Autodesk Fusion 360 part; units mm, degrees
note: some values were not read from the file. Set by a fixed rule: which sketch regions a step uses.
(part 15 of 20)
  spline S84 degree 5 poles (-28.7753, 3.9508) (-28.7754, 3.9508) (-28.7756, 3.9508) (-28.7759, 3.9509) (-28.7764, 3.9509) (-28.7772, 3.951) (-28.778, 3.9511) (-28.779, 3.9512) (-28.7801, 3.9514) (-28.7813, 3.9515) (-28.7826, 3.9517) (-28.784, 3.9518) (-28.7855, 3.952) (-28.7871, 3.9522) (-28.7889, 3.9523) (-28.7907, 3.9525) (-28.7926, 3.9527) (-28.7946, 3.9529) (-28.7968, 3.9531) (-28.799, 3.9534) (-28.8013, 3.9536) (-28.8037, 3.9538) (-28.8063, 3.954) (-28.8089, 3.9543) (-28.8116, 3.9545) (-28.8144, 3.9547) (-28.8172, 3.955) (-28.8202, 3.9552) (-28.8233, 3.9555) (-28.8264, 3.9557) (-28.8297, 3.9559) (-28.833, 3.9562) (-28.8364, 3.9564) (-28.8399, 3.9567) (-28.8435, 3.9569) (-28.8472, 3.9572) (-28.8509, 3.9574) (-28.8547, 3.9577) (-28.8586, 3.9579) (-28.8626, 3.9581) (-28.8667, 3.9584) (-28.8709, 3.9586) (-28.8751, 3.9588) (-28.8794, 3.959) (-28.8838, 3.9593) (-28.8882, 3.9595) (-28.8928, 3.9597) (-28.8974, 3.9599) (-28.9021, 3.9601) (-28.9068, 3.9603) (-28.9117, 3.9605) (-28.9166, 3.9607) (-28.9215, 3.9609) (-28.9266, 3.961) (-28.9317, 3.9612) (-28.9369, 3.9614) (-28.9422, 3.9615) (-28.9475, 3.9617) (-28.9529, 3.9618) (-28.9584, 3.962) (-28.9639, 3.9621) (-28.9695, 3.9622) (-28.9752, 3.9623) (-28.9809, 3.9624) (-28.9867, 3.9625) (-28.9926, 3.9626) (-28.9985, 3.9627) (-29.0045, 3.9627) (-29.0106, 3.9628) (-29.0167, 3.9629) (-29.0229, 3.9629) (-29.0291, 3.9629) (-29.0355, 3.9629) (-29.0418, 3.963) (-29.0483, 3.963) (-29.0548, 3.9629) (-29.0613, 3.9629) (-29.068, 3.9629) (-29.0746, 3.9628) (-29.0814, 3.9628) (-29.0882, 3.9627) (-29.095, 3.9626) (-29.1019, 3.9626) (-29.1089, 3.9625) (-29.1159, 3.9623) (-29.123, 3.9622) (-29.1302, 3.9621) (-29.1374, 3.9619) (-29.1446, 3.9618) (-29.1519, 3.9616) (-29.1593, 3.9614) (-29.1667, 3.9612) (-29.1742, 3.961) (-29.1817, 3.9607) (-29.1893, 3.9605) (-29.197, 3.9603) (-29.2047, 3.96) (-29.2124, 3.9597) (-29.2202, 3.9594) (-29.2281, 3.9591) (-29.236, 3.9588) (-29.2439, 3.9584) (-29.2519, 3.9581) (-29.26, 3.9577) (-29.2681, 3.9573) (-29.2763, 3.9569) (-29.2845, 3.9565) (-29.2927, 3.9561) (-29.301, 3.9556) (-29.3094, 3.9552) (-29.3178, 3.9547) (-29.3263, 3.9542) (-29.3348, 3.9537) (-29.3433, 3.9532) (-29.3519, 3.9526) (-29.3606, 3.9521) (-29.3693, 3.9515) (-29.378, 3.9509) (-29.3868, 3.9503) (-29.3957, 3.9497) (-29.4045, 3.9491) (-29.4135, 3.9484) (-29.4225, 3.9478) (-29.4315, 3.9471) (-29.4406, 3.9464) (-29.4497, 3.9457) (-29.4588, 3.9449) (-29.468, 3.9442) (-29.4773, 3.9434) (-29.4866, 3.9426) (-29.4959, 3.9418) (-29.5053, 3.941) (-29.5147, 3.9402) (-29.5242, 3.9393) (-29.5337, 3.9384) (-29.5433, 3.9375) (-29.5529, 3.9366) (-29.5625, 3.9357) (-29.5722, 3.9348) (-29.5819, 3.9338) (-29.5917, 3.9328) (-29.6015, 3.9318) (-29.6113, 3.9308) (-29.6212, 3.9297) (-29.6312, 3.9287) (-29.6411, 3.9276) (-29.6512, 3.9265) (-29.6612, 3.9254) (-29.6713, 3.9243) (-29.6814, 3.9231) (-29.6916, 3.922) (-29.7018, 3.9208) (-29.7121, 3.9196) (-29.7224, 3.9183) (-29.7327, 3.9171) (-29.7431, 3.9158) (-29.7535, 3.9145) (-29.764, 3.9132) (-29.7744, 3.9119) (-29.785, 3.9106) (-29.7955, 3.9092) (-29.8061, 3.9078) (-29.8168, 3.9064) (-29.8274, 3.905) (-29.8382, 3.9035) (-29.8489, 3.9021) (-29.8597, 3.9006) (-29.8705, 3.8991) (-29.8814, 3.8976) (-29.8923, 3.896) (-29.9032, 3.8945) (-29.9142, 3.8929) (-29.9252, 3.8913) (-29.9362, 3.8896) (-29.9473, 3.888) (-29.9584, 3.8863) (-29.9696, 3.8846) (-29.9807, 3.8829) (-29.992, 3.8812) (-30.0032, 3.8795) (-30.0145, 3.8777) (-30.0258, 3.8759) (-30.0372, 3.8741) (-30.0486, 3.8722) (-30.06, 3.8704) (-30.0714, 3.8685) (-30.0829, 3.8666) (-30.0944, 3.8647) (-30.106, 3.8628) (-30.1176, 3.8608) (-30.1292, 3.8588) (-30.1409, 3.8568) (-30.1525, 3.8548) (-30.1643, 3.8527) (-30.176, 3.8507) (-30.1878, 3.8486) (-30.1996, 3.8464) (-30.2115, 3.8443) (-30.2233, 3.8422) (-30.2353, 3.84) (-30.2472, 3.8378) (-30.2592, 3.8356) (-30.2712, 3.8333) (-30.2832, 3.831) (-30.2953, 3.8288) (-30.3074, 3.8264) (-30.3195, 3.8241) (-30.3317, 3.8217) (-30.3439, 3.8194) (-30.3561, 3.817) (-30.3683, 3.8145) (-30.3806, 3.8121) (-30.3929, 3.8096) (-30.4053, 3.8071) (-30.4176, 3.8046) (-30.43, 3.8021) (-30.4424, 3.7995) (-30.4549, 3.797) (-30.4674, 3.7943) (-30.4799, 3.7917) (-30.4924, 3.7891) (-30.505, 3.7864) (-30.5176, 3.7837) (-30.5302, 3.781) (-30.5429, 3.7782) (-30.5556, 3.7755) (-30.5683, 3.7727) (-30.581, 3.7699) (-30.5938, 3.767) (-30.6066, 3.7642) (-30.6194, 3.7613) (-30.6323, 3.7584) (-30.6451, 3.7555) (-30.658, 3.7525) (-30.671, 3.7496) (-30.6839, 3.7466) (-30.6969, 3.7435) (-30.7099, 3.7405) (-30.723, 3.7374) (-30.736, 3.7343) (-30.7491, 3.7312) (-30.7596, 3.7287) (-30.7675, 3.7268) (-30.7728, 3.7256) (-30.7754, 3.7249) knots 0 0 0 0 0 0 0.00416667 0.00833333 0.0125 0.01666667 0.02083333 0.025 0.02916667 0.03333333 0.0375 0.04166667 0.04583333 0.05 0.05416667 0.05833333 0.0625 0.06666667 0.07083333 0.075 0.07916667 0.08333333 0.0875 0.09166667 0.09583333 0.1 0.10416667 0.10833333 0.1125 0.11666667 0.12083333 0.125 0.12916667 0.13333333 0.1375 0.14166667 0.14583333 0.15 0.15416667 0.15833333 0.1625 0.16666667 0.17083333 0.175 0.17916667 0.18333333 0.1875 0.19166667 0.19583333 0.2 0.20416667 0.20833333 0.2125 0.21666667 0.22083333 0.225 0.22916667 0.23333333 0.2375 0.24166667 0.24583333 0.25 0.25416667 0.25833333 0.2625 0.26666667 0.27083333 0.275 0.27916667 0.28333333 0.2875 0.29166667 0.29583333 0.3 0.30416667 0.30833333 0.3125 0.31666667 0.32083333 0.325 0.32916667 0.33333333 0.3375 0.34166667 0.34583333 0.35 0.35416667 0.35833333 0.3625 0.36666667 0.37083333 0.375 0.37916667 0.38333333 0.3875 0.39166667 0.39583333 0.4 0.40416667 0.40833333 0.4125 0.41666667 0.42083333 0.425 0.42916667 0.43333333 0.4375 0.44166667 0.44583333 0.45 0.45416667 0.45833333 0.4625 0.46666667 0.47083333 0.475 0.47916667 0.48333333 0.4875 0.49166667 0.49583333 0.5 0.50416667 0.50833333 0.5125 0.51666667 0.52083333 0.525 0.52916667 0.53333333 0.5375 0.54166667 0.54583333 0.55 0.55416667 0.55833333 0.5625 0.56666667 0.57083333 0.575 0.57916667 0.58333333 0.5875 0.59166667 0.59583333 0.6 0.60416667 0.60833333 0.6125 0.61666667 0.62083333 0.625 0.62916667 0.63333333 0.6375 0.64166667 0.64583333 0.65 0.65416667 0.65833333 0.6625 0.66666667 0.67083333 0.675 0.67916667 0.68333333 0.6875 0.69166667 0.69583333 0.7 0.70416667 0.70833333 0.7125 0.71666667 0.72083333 0.725 0.72916667 0.73333333 0.7375 0.74166667 0.74583333 0.75 0.75416667 0.75833333 0.7625 0.76666667 0.77083333 0.775 0.77916667 0.78333333 0.7875 0.79166667 0.79583333 0.8 0.80416667 0.80833333 0.8125 0.81666667 0.82083333 0.825 0.82916667 0.83333333 0.8375 0.84166667 0.84583333 0.85 0.85416667 0.85833333 0.8625 0.86666667 0.87083333 0.875 0.87916667 0.88333333 0.8875 0.89166667 0.89583333 0.9 0.90416667 0.90833333 0.9125 0.91666667 0.92083333 0.925 0.92916667 0.93333333 0.9375 0.94166667 0.94583333 0.95 0.95416667 0.95833333 0.9625 0.96666667 0.97083333 0.975 0.97916667 0.98333333 0.9875 0.99166667 0.99583333 1 1 1 1 1 1
  arc A83 (-30.9962, 0.4876) -> (-30.9962, -0.4876) centre (0, 0) ccw
  line L180 (-27.8945, 8.0948) -> (-27.8937, 8.0945)
  spline S85 degree 5 poles (12.1618, 28.5147) (12.16, 28.5128) (12.1562, 28.5089) (12.1506, 28.503) (12.1432, 28.4951) (12.134, 28.4854) (12.1248, 28.4756) (12.1156, 28.4658) (12.1065, 28.4561) (12.0973, 28.4464) (12.0883, 28.4366) (12.0792, 28.4269) (12.0702, 28.4172) (12.0613, 28.4075) (12.0523, 28.3978) (12.0434, 28.3882) (12.0345, 28.3785) (12.0257, 28.3689) (12.0169, 28.3593) (12.0081, 28.3496) (11.9994, 28.34) (11.9907, 28.3305) (11.982, 28.3209) (11.9734, 28.3113) (11.9648, 28.3018) (11.9562, 28.2922) (11.9477, 28.2827) (11.9392, 28.2732) (11.9307, 28.2637) (11.9223, 28.2542) (11.9139, 28.2447) (11.9055, 28.2353) (11.8972, 28.2259) (11.8889, 28.2164) (11.8807, 28.207) (11.8724, 28.1976) (11.8643, 28.1882) (11.8561, 28.1789) (11.848, 28.1695) (11.8399, 28.1602) (11.8318, 28.1509) (11.8238, 28.1416) (11.8158, 28.1323) (11.8079, 28.123) (11.8, 28.1137) (11.7921, 28.1045) (11.7843, 28.0953) (11.7765, 28.0861) (11.7687, 28.0769) (11.7609, 28.0677) (11.7532, 28.0585) (11.7456, 28.0494) (11.7379, 28.0403) (11.7303, 28.0312) (11.7228, 28.0221) (11.7153, 28.013) (11.7078, 28.0039) (11.7003, 27.9949) (11.6929, 27.9859) (11.6855, 27.9769) (11.6781, 27.9679) (11.6708, 27.9589) (11.6635, 27.95) (11.6563, 27.9411) (11.6491, 27.9322) (11.6419, 27.9233) (11.6348, 27.9144) (11.6276, 27.9055) (11.6206, 27.8967) (11.6135, 27.8879) (11.6065, 27.8791) (11.5996, 27.8704) (11.5927, 27.8616) (11.5858, 27.8529) (11.5789, 27.8442) (11.5721, 27.8355) (11.5653, 27.8268) (11.5585, 27.8182) (11.5518, 27.8096) (11.5452, 27.801) (11.5385, 27.7924) (11.5319, 27.7838) (11.5253, 27.7753) (11.5188, 27.7668) (11.5123, 27.7583) (11.5058, 27.7498) (11.4994, 27.7414) (11.493, 27.733) (11.4867, 27.7246) (11.4803, 27.7162) (11.4741, 27.7078) (11.4678, 27.6995) (11.4616, 27.6912) (11.4554, 27.6829) (11.4493, 27.6747) (11.4432, 27.6665) (11.4371, 27.6582) (11.4311, 27.6501) (11.4251, 27.6419) (11.4192, 27.6338) (11.4132, 27.6257) (11.4074, 27.6176) (11.4015, 27.6096) (11.3957, 27.6015) (11.3899, 27.5936) (11.3842, 27.5856) (11.3785, 27.5776) (11.3728, 27.5697) (11.3672, 27.5618) (11.3616, 27.554) (11.3561, 27.5462) (11.3506, 27.5384) (11.3451, 27.5306) (11.3396, 27.5228) (11.3342, 27.5151) (11.3289, 27.5074) (11.3235, 27.4998) (11.3183, 27.4922) (11.313, 27.4846) (11.3078, 27.477) (11.3026, 27.4695) (11.2975, 27.462) (11.2924, 27.4545) (11.2873, 27.447) (11.2823, 27.4396) (11.2773, 27.4323) (11.2723, 27.4249) (11.2674, 27.4176) (11.2625, 27.4103) (11.2577, 27.4031) (11.2529, 27.3958) (11.2481, 27.3887) (11.2434, 27.3815) (11.2387, 27.3744) (11.234, 27.3673) (11.2294, 27.3603) (11.2248, 27.3533) (11.2203, 27.3463) (11.2158, 27.3393) (11.2113, 27.3324) (11.2069, 27.3256) (11.2025, 27.3187) (11.1982, 27.3119) (11.1939, 27.3052) (11.1896, 27.2985) (11.1854, 27.2918) (11.1812, 27.2851) (11.177, 27.2785) (11.1729, 27.272) (11.1688, 27.2654) (11.1648, 27.259) (11.1608, 27.2525) (11.1568, 27.2461) (11.1529, 27.2397) (11.149, 27.2334) (11.1451, 27.2271) (11.1413, 27.2209) (11.1376, 27.2147) (11.1338, 27.2085) (11.1301, 27.2024) (11.1265, 27.1963) (11.1229, 27.1903) (11.1193, 27.1843) (11.1158, 27.1784) (11.1123, 27.1725) (11.1088, 27.1666) (11.1054, 27.1608) (11.102, 27.155) (11.0987, 27.1493) (11.0954, 27.1436) (11.0921, 27.138) (11.0889, 27.1324) (11.0857, 27.1269) (11.0826, 27.1214) (11.0795, 27.116) (11.0764, 27.1106) (11.0734, 27.1053) (11.0704, 27.1) (11.0675, 27.0948) (11.0646, 27.0896) (11.0617, 27.0845) (11.0589, 27.0794) (11.0561, 27.0744) (11.0534, 27.0694) (11.0507, 27.0645) (11.048, 27.0597) (11.0454, 27.0549) (11.0428, 27.0501) (11.0403, 27.0454) (11.0378, 27.0408) (11.0353, 27.0362) (11.0329, 27.0317) (11.0306, 27.0272) (11.0282, 27.0228) (11.0259, 27.0185) (11.0237, 27.0142) (11.0215, 27.01) (11.0193, 27.0058) (11.0172, 27.0017) (11.0151, 26.9977) (11.0131, 26.9937) (11.0111, 26.9898) (11.0091, 26.986) (11.0072, 26.9822) (11.0053, 26.9785) (11.0035, 26.9748) (11.0017, 26.9713) (10.9999, 26.9678) (10.9982, 26.9643) (10.9966, 26.961) (10.9949, 26.9577) (10.9934, 26.9544) (10.9918, 26.9513) (10.9903, 26.9482) (10.9889, 26.9452) (10.9875, 26.9423) (10.9861, 26.9394) (10.9848, 26.9366) (10.9835, 26.9339) (10.9823, 26.9313) (10.9811, 26.9288) (10.9799, 26.9263) (10.9788, 26.924) (10.9778, 26.9217) (10.9768, 26.9195) (10.9758, 26.9173) (10.9749, 26.9153) (10.974, 26.9134) (10.9731, 26.9115) (10.9724, 26.9097) (10.9716, 26.908) (10.9709, 26.9065) (10.9702, 26.905) (10.9696, 26.9036) (10.9691, 26.9023) (10.9685, 26.9011) (10.9681, 26.9) (10.9676, 26.899) (10.9672, 26.8981) (10.9669, 26.8973) (10.9666, 26.8966) (10.9664, 26.8961) (10.9663, 26.8958) (10.9662, 26.8956) (10.9662, 26.8955) knots -1 -1 -1 -1 -1 -1 -0.99583333 -0.99166667 -0.9875 -0.98333333 -0.97916667 -0.975 -0.97083333 -0.96666667 -0.9625 -0.95833333 -0.95416667 -0.95 -0.94583333 -0.94166667 -0.9375 -0.93333333 -0.92916667 -0.925 -0.92083333 -0.91666667 -0.9125 -0.90833333 -0.90416667 -0.9 -0.89583333 -0.89166667 -0.8875 -0.88333333 -0.87916667 -0.875 -0.87083333 -0.86666667 -0.8625 -0.85833333 -0.85416667 -0.85 -0.84583333 -0.84166667 -0.8375 -0.83333333 -0.82916667 -0.825 -0.82083333 -0.81666667 -0.8125 -0.80833333 -0.80416667 -0.8 -0.79583333 -0.79166667 -0.7875 -0.78333333 -0.77916667 -0.775 -0.77083333 -0.76666667 -0.7625 -0.75833333 -0.75416667 -0.75 -0.74583333 -0.74166667 -0.7375 -0.73333333 -0.72916667 -0.725 -0.72083333 -0.71666667 -0.7125 -0.70833333 -0.70416667 -0.7 -0.69583333 -0.69166667 -0.6875 -0.68333333 -0.67916667 -0.675 -0.67083333 -0.66666667 -0.6625 -0.65833333 -0.65416667 -0.65 -0.64583333 -0.64166667 -0.6375 -0.63333333 -0.62916667 -0.625 -0.62083333 -0.61666667 -0.6125 -0.60833333 -0.60416667 -0.6 -0.59583333 -0.59166667 -0.5875 -0.58333333 -0.57916667 -0.575 -0.57083333 -0.56666667 -0.5625 -0.55833333 -0.55416667 -0.55 -0.54583333 -0.54166667 -0.5375 -0.53333333 -0.52916667 -0.525 -0.52083333 -0.51666667 -0.5125 -0.50833333 -0.50416667 -0.5 -0.49583333 -0.49166667 -0.4875 -0.48333333 -0.47916667 -0.475 -0.47083333 -0.46666667 -0.4625 -0.45833333 -0.45416667 -0.45 -0.44583333 -0.44166667 -0.4375 -0.43333333 -0.42916667 -0.425 -0.42083333 -0.41666667 -0.4125 -0.40833333 -0.40416667 -0.4 -0.39583333 -0.39166667 -0.3875 -0.38333333 -0.37916667 -0.375 -0.37083333 -0.36666667 -0.3625 -0.35833333 -0.35416667 -0.35 -0.34583333 -0.34166667 -0.3375 -0.33333333 -0.32916667 -0.325 -0.32083333 -0.31666667 -0.3125 -0.30833333 -0.30416667 -0.3 -0.29583333 -0.29166667 -0.2875 -0.28333333 -0.27916667 -0.275 -0.27083333 -0.26666667 -0.2625 -0.25833333 -0.25416667 -0.25 -0.24583333 -0.24166667 -0.2375 -0.23333333 -0.22916667 -0.225 -0.22083333 -0.21666667 -0.2125 -0.20833333 -0.20416667 -0.2 -0.19583333 -0.19166667 -0.1875 -0.18333333 -0.17916667 -0.175 -0.17083333 -0.16666667 -0.1625 -0.15833333 -0.15416667 -0.15 -0.14583333 -0.14166667 -0.1375 -0.13333333 -0.12916667 -0.125 -0.12083333 -0.11666667 -0.1125 -0.10833333 -0.10416667 -0.1 -0.09583333 -0.09166667 -0.0875 -0.08333333 -0.07916667 -0.075 -0.07083333 -0.06666667 -0.0625 -0.05833333 -0.05416667 -0.05 -0.04583333 -0.04166667 -0.0375 -0.03333333 -0.02916667 -0.025 -0.02083333 -0.01666667 -0.0125 -0.00833333 -0.00416667 0 0 0 0 0 0
  arc A84 (10.0421, 29.3284) -> (9.1146, 29.6298) centre (0, 0) ccw
  arc A85 (10.8547, 26.6221) -> (9.7471, 27.0473) centre (0, 0) ccw
  line L181 (-28.7745, 3.9507) -> (-28.7753, 3.9508)
  line L182 (-28.9671, 2.1182) -> (-28.6734, 2.0967)
  arc A86 (13.0527, 28.1181) -> (12.1618, 28.5147) centre (0, 0) ccw
  arc A87 (13.578, 25.3417) -> (12.5209, 25.8803) centre (0, 0) ccw
  line L183 (-28.4828, 3.9106) -> (-28.7745, 3.9507)
  arc A88 (-30.7754, 3.7249) -> (-30.8773, 2.755) centre (0, 0) ccw
  spline S86 degree 5 poles (-29.0307, 0.9213) (-29.0307, 0.9213) (-29.0309, 0.9213) (-29.0313, 0.9213) (-29.0318, 0.9213) (-29.0325, 0.9213) (-29.0334, 0.9213) (-29.0344, 0.9214) (-29.0355, 0.9214) (-29.0367, 0.9214) (-29.038, 0.9214) (-29.0394, 0.9214) (-29.0409, 0.9214) (-29.0425, 0.9214) (-29.0443, 0.9214) (-29.0461, 0.9214) (-29.0481, 0.9214) (-29.0501, 0.9214) (-29.0522, 0.9214) (-29.0545, 0.9214) (-29.0568, 0.9214) (-29.0592, 0.9213) (-29.0618, 0.9213) (-29.0644, 0.9212) (-29.0671, 0.9212) (-29.0699, 0.9211) (-29.0728, 0.9211) (-29.0758, 0.921) (-29.0788, 0.9209) (-29.082, 0.9208) (-29.0852, 0.9208) (-29.0886, 0.9206) (-29.092, 0.9205) (-29.0955, 0.9204) (-29.0991, 0.9203) (-29.1028, 0.9201) (-29.1065, 0.92) (-29.1103, 0.9198) (-29.1143, 0.9197) (-29.1183, 0.9195) (-29.1223, 0.9193) (-29.1265, 0.9191) (-29.1307, 0.9189) (-29.135, 0.9186) (-29.1394, 0.9184) (-29.1439, 0.9182) (-29.1484, 0.9179) (-29.153, 0.9176) (-29.1577, 0.9173) (-29.1624, 0.917) (-29.1673, 0.9167) (-29.1722, 0.9164) (-29.1771, 0.9161) (-29.1822, 0.9157) (-29.1873, 0.9153) (-29.1925, 0.915) (-29.1977, 0.9146) (-29.203, 0.9141) (-29.2084, 0.9137) (-29.2139, 0.9133) (-29.2194, 0.9128) (-29.225, 0.9124) (-29.2306, 0.9119) (-29.2363, 0.9114) (-29.2421, 0.9109) (-29.248, 0.9103) (-29.2539, 0.9098) (-29.2599, 0.9092) (-29.2659, 0.9087) (-29.272, 0.9081) (-29.2781, 0.9075) (-29.2844, 0.9068) (-29.2906, 0.9062) (-29.297, 0.9055) (-29.3034, 0.9049) (-29.3099, 0.9042) (-29.3164, 0.9035) (-29.323, 0.9027) (-29.3296, 0.902) (-29.3363, 0.9012) (-29.343, 0.9005) (-29.3498, 0.8997) (-29.3567, 0.8989) (-29.3636, 0.898) (-29.3706, 0.8972) (-29.3777, 0.8963) (-29.3847, 0.8954) (-29.3919, 0.8945) (-29.3991, 0.8936) (-29.4063, 0.8927) (-29.4137, 0.8917) (-29.421, 0.8907) (-29.4284, 0.8897) (-29.4359, 0.8887) (-29.4434, 0.8877) (-29.451, 0.8866) (-29.4586, 0.8856) (-29.4663, 0.8845) (-29.474, 0.8834) (-29.4818, 0.8822) (-29.4896, 0.8811) (-29.4975, 0.8799) (-29.5054, 0.8787) (-29.5134, 0.8775) (-29.5214, 0.8763) (-29.5295, 0.875) (-29.5376, 0.8738) (-29.5458, 0.8725) (-29.554, 0.8712) (-29.5623, 0.8698) (-29.5706, 0.8685) (-29.5789, 0.8671) (-29.5873, 0.8657) (-29.5958, 0.8643) (-29.6043, 0.8629) (-29.6128, 0.8614) (-29.6214, 0.86) (-29.6301, 0.8585) (-29.6388, 0.8569) (-29.6475, 0.8554) (-29.6563, 0.8538) (-29.6651, 0.8523) (-29.6739, 0.8507) (-29.6828, 0.849) (-29.6918, 0.8474) (-29.7008, 0.8457) (-29.7098, 0.844) (-29.7189, 0.8423) (-29.728, 0.8406) (-29.7372, 0.8388) (-29.7464, 0.8371) (-29.7556, 0.8353) (-29.7649, 0.8334) (-29.7742, 0.8316) (-29.7836, 0.8297) (-29.793, 0.8279) (-29.8025, 0.8259) (-29.812, 0.824) (-29.8215, 0.8221) (-29.8311, 0.8201) (-29.8407, 0.8181) (-29.8503, 0.8161) (-29.86, 0.814) (-29.8697, 0.812) (-29.8795, 0.8099) (-29.8893, 0.8078) (-29.8992, 0.8056) (-29.909, 0.8035) (-29.919, 0.8013) (-29.9289, 0.7991) (-29.9389, 0.7969) (-29.949, 0.7946) (-29.959, 0.7923) (-29.9691, 0.79) (-29.9793, 0.7877) (-29.9895, 0.7854) (-29.9997, 0.783) (-30.0099, 0.7806) (-30.0202, 0.7782) (-30.0306, 0.7758) (-30.0409, 0.7733) (-30.0513, 0.7708) (-30.0618, 0.7683) (-30.0722, 0.7658) (-30.0827, 0.7632) (-30.0933, 0.7606) (-30.1038, 0.758) (-30.1145, 0.7554) (-30.1251, 0.7528) (-30.1358, 0.7501) (-30.1465, 0.7474) (-30.1572, 0.7447) (-30.168, 0.7419) (-30.1788, 0.7391) (-30.1897, 0.7364) (-30.2005, 0.7335) (-30.2114, 0.7307) (-30.2224, 0.7278) (-30.2334, 0.7249) (-30.2444, 0.722) (-30.2554, 0.7191) (-30.2665, 0.7161) (-30.2776, 0.7131) (-30.2887, 0.7101) (-30.2999, 0.7071) (-30.3111, 0.704) (-30.3223, 0.7009) (-30.3336, 0.6978) (-30.3448, 0.6947) (-30.3562, 0.6915) (-30.3675, 0.6883) (-30.3789, 0.6851) (-30.3903, 0.6819) (-30.4017, 0.6786) (-30.4132, 0.6753) (-30.4247, 0.672) (-30.4362, 0.6687) (-30.4478, 0.6653) (-30.4594, 0.6619) (-30.471, 0.6585) (-30.4827, 0.6551) (-30.4943, 0.6516) (-30.506, 0.6481) (-30.5178, 0.6446) (-30.5295, 0.6411) (-30.5413, 0.6375) (-30.5531, 0.6339) (-30.565, 0.6303) (-30.5769, 0.6267) (-30.5888, 0.623) (-30.6007, 0.6193) (-30.6126, 0.6156) (-30.6246, 0.6118) (-30.6366, 0.6081) (-30.6487, 0.6043) (-30.6607, 0.6005) (-30.6728, 0.5966) (-30.685, 0.5927) (-30.6971, 0.5889) (-30.7093, 0.5849) (-30.7215, 0.581) (-30.7337, 0.577) (-30.7459, 0.573) (-30.7582, 0.569) (-30.7705, 0.5649) (-30.7828, 0.5609) (-30.7952, 0.5568) (-30.8076, 0.5526) (-30.82, 0.5485) (-30.8324, 0.5443) (-30.8448, 0.5401) (-30.8573, 0.5359) (-30.8698, 0.5316) (-30.8823, 0.5273) (-30.8949, 0.523) (-30.9075, 0.5187) (-30.9201, 0.5143) (-30.9327, 0.5099) (-30.9453, 0.5055) (-30.958, 0.5011) (-30.9707, 0.4966) (-30.9809, 0.493) (-30.9885, 0.4903) (-30.9936, 0.4885) (-30.9962, 0.4876) knots 0 0 0 0 0 0 0.00416667 0.00833333 0.0125 0.01666667 0.02083333 0.025 0.02916667 0.03333333 0.0375 0.04166667 0.04583333 0.05 0.05416667 0.05833333 0.0625 0.06666667 0.07083333 0.075 0.07916667 0.08333333 0.0875 0.09166667 0.09583333 0.1 0.10416667 0.10833333 0.1125 0.11666667 0.12083333 0.125 0.12916667 0.13333333 0.1375 0.14166667 0.14583333 0.15 0.15416667 0.15833333 0.1625 0.16666667 0.17083333 0.175 0.17916667 0.18333333 0.1875 0.19166667 0.19583333 0.2 0.20416667 0.20833333 0.2125 0.21666667 0.22083333 0.225 0.22916667 0.23333333 0.2375 0.24166667 0.24583333 0.25 0.25416667 0.25833333 0.2625 0.26666667 0.27083333 0.275 0.27916667 0.28333333 0.2875 0.29166667 0.29583333 0.3 0.30416667 0.30833333 0.3125 0.31666667 0.32083333 0.325 0.32916667 0.33333333 0.3375 0.34166667 0.34583333 0.35 0.35416667 0.35833333 0.3625 0.36666667 0.37083333 0.375 0.37916667 0.38333333 0.3875 0.39166667 0.39583333 0.4 0.40416667 0.40833333 0.4125 0.41666667 0.42083333 0.425 0.42916667 0.43333333 0.4375 0.44166667 0.44583333 0.45 0.45416667 0.45833333 0.4625 0.46666667 0.47083333 0.475 0.47916667 0.48333333 0.4875 0.49166667 0.49583333 0.5 0.50416667 0.50833333 0.5125 0.51666667 0.52083333 0.525 0.52916667 0.53333333 0.5375 0.54166667 0.54583333 0.55 0.55416667 0.55833333 0.5625 0.56666667 0.57083333 0.575 0.57916667 0.58333333 0.5875 0.59166667 0.59583333 0.6 0.60416667 0.60833333 0.6125 0.61666667 0.62083333 0.625 0.62916667 0.63333333 0.6375 0.64166667 0.64583333 0.65 0.65416667 0.65833333 0.6625 0.66666667 0.67083333 0.675 0.67916667 0.68333333 0.6875 0.69166667 0.69583333 0.7 0.70416667 0.70833333 0.7125 0.71666667 0.72083333 0.725 0.72916667 0.73333333 0.7375 0.74166667 0.74583333 0.75 0.75416667 0.75833333 0.7625 0.76666667 0.77083333 0.775 0.77916667 0.78333333 0.7875 0.79166667 0.79583333 0.8 0.80416667 0.80833333 0.8125 0.81666667 0.82083333 0.825 0.82916667 0.83333333 0.8375 0.84166667 0.84583333 0.85 0.85416667 0.85833333 0.8625 0.86666667 0.87083333 0.875 0.87916667 0.88333333 0.8875 0.89166667 0.89583333 0.9 0.90416667 0.90833333 0.9125 0.91666667 0.92083333 0.925 0.92916667 0.93333333 0.9375 0.94166667 0.94583333 0.95 0.95416667 0.95833333 0.9625 0.96666667 0.97083333 0.975 0.97916667 0.98333333 0.9875 0.99166667 0.99583333 1 1 1 1 1 1
  spline S87 degree 5 poles (12.6495, 26.1461) (12.6495, 26.1462) (12.6496, 26.1464) (12.6497, 26.1467) (12.65, 26.1471) (12.6503, 26.1478) (12.6506, 26.1486) (12.651, 26.1495) (12.6515, 26.1504) (12.652, 26.1515) (12.6526, 26.1527) (12.6531, 26.154) (12.6538, 26.1554) (12.6544, 26.1569) (12.6551, 26.1585) (12.6559, 26.1602) (12.6567, 26.1619) (12.6575, 26.1638) (12.6583, 26.1658) (12.6592, 26.1678) (12.6602, 26.17) (12.6611, 26.1722) (12.6621, 26.1745) (12.6631, 26.1769) (12.6642, 26.1794) (12.6653, 26.182) (12.6664, 26.1847) (12.6676, 26.1874) (12.6687, 26.1903) (12.6699, 26.1932) (12.6712, 26.1962) (12.6724, 26.1993) (12.6737, 26.2024) (12.675, 26.2057) (12.6764, 26.209) (12.6778, 26.2124) (12.6791, 26.2159) (12.6806, 26.2195) (12.682, 26.2231) (12.6834, 26.2269) (12.6849, 26.2307) (12.6864, 26.2345) (12.688, 26.2385) (12.6895, 26.2425) (12.6911, 26.2466) (12.6927, 26.2508) (12.6943, 26.255) (12.6959, 26.2594) (12.6975, 26.2638) (12.6992, 26.2682) (12.7009, 26.2728) (12.7026, 26.2774) (12.7043, 26.282) (12.706, 26.2868) (12.7077, 26.2916) (12.7095, 26.2965) (12.7113, 26.3015) (12.7131, 26.3065) (12.7149, 26.3116) (12.7167, 26.3167) (12.7185, 26.322) (12.7204, 26.3273) (12.7222, 26.3326) (12.7241, 26.338) (12.726, 26.3435) (12.7279, 26.3491) (12.7298, 26.3547) (12.7317, 26.3604) (12.7336, 26.3661) (12.7356, 26.3719) (12.7375, 26.3778) (12.7395, 26.3837) (12.7414, 26.3897) (12.7434, 26.3958) (12.7454, 26.4019) (12.7474, 26.4081) (12.7494, 26.4144) (12.7514, 26.4207) (12.7534, 26.427) (12.7555, 26.4335) (12.7575, 26.4399) (12.7596, 26.4465) (12.7616, 26.4531) (12.7637, 26.4598) (12.7657, 26.4665) (12.7678, 26.4733) (12.7699, 26.4801) (12.772, 26.487) (12.774, 26.4939) (12.7761, 26.5009) (12.7782, 26.508) (12.7803, 26.5151) (12.7824, 26.5223) (12.7845, 26.5296) (12.7867, 26.5368) (12.7888, 26.5442) (12.7909, 26.5516) (12.793, 26.559) (12.7952, 26.5665) (12.7973, 26.5741) (12.7994, 26.5817) (12.8016, 26.5894) (12.8037, 26.5971) (12.8058, 26.6049) (12.808, 26.6127) (12.8101, 26.6206) (12.8123, 26.6286) (12.8144, 26.6365) (12.8166, 26.6446) (12.8187, 26.6527) (12.8208, 26.6608) (12.823, 26.669) (12.8251, 26.6773) (12.8273, 26.6856) (12.8294, 26.6939) (12.8316, 26.7023) (12.8337, 26.7108) (12.8359, 26.7193) (12.838, 26.7278) (12.8402, 26.7364) (12.8423, 26.7451) (12.8445, 26.7537) (12.8466, 26.7625) (12.8487, 26.7713) (12.8509, 26.7801) (12.853, 26.789) (12.8551, 26.798) (12.8573, 26.8069) (12.8594, 26.816) (12.8615, 26.8251) (12.8636, 26.8342) (12.8658, 26.8434) (12.8679, 26.8526) (12.87, 26.8619) (12.8721, 26.8712) (12.8742, 26.8806) (12.8763, 26.89) (12.8784, 26.8994) (12.8805, 26.9089) (12.8826, 26.9185) (12.8847, 26.9281) (12.8867, 26.9377) (12.8888, 26.9474) (12.8909, 26.9571) (12.8929, 26.9669) (12.895, 26.9767) (12.8971, 26.9866) (12.8991, 26.9965) (12.9011, 27.0064) (12.9032, 27.0164) (12.9052, 27.0265) (12.9072, 27.0365) (12.9093, 27.0467) (12.9113, 27.0568) (12.9133, 27.0671) (12.9153, 27.0773) (12.9173, 27.0876) (12.9193, 27.0979) (12.9213, 27.1083) (12.9232, 27.1188) (12.9252, 27.1292) (12.9272, 27.1397) (12.9291, 27.1503) (12.9311, 27.1609) (12.933, 27.1715) (12.9349, 27.1822) (12.9368, 27.1929) (12.9388, 27.2037) (12.9407, 27.2145) (12.9426, 27.2253) (12.9445, 27.2362) (12.9463, 27.2471) (12.9482, 27.2581) (12.9501, 27.2691) (12.9519, 27.2801) (12.9538, 27.2912) (12.9556, 27.3023) (12.9574, 27.3135) (12.9593, 27.3247) (12.9611, 27.3359) (12.9629, 27.3472) (12.9647, 27.3585) (12.9665, 27.3699) (12.9682, 27.3813) (12.97, 27.3927) (12.9718, 27.4042) (12.9735, 27.4157) (12.9752, 27.4273) (12.977, 27.4388) (12.9787, 27.4505) (12.9804, 27.4621) (12.9821, 27.4738) (12.9838, 27.4856) (12.9854, 27.4974) (12.9871, 27.5092) (12.9887, 27.521) (12.9904, 27.5329) (12.992, 27.5449) (12.9936, 27.5568) (12.9952, 27.5688) (12.9968, 27.5809) (12.9984, 27.5929) (13, 27.605) (13.0016, 27.6172) (13.0031, 27.6294) (13.0047, 27.6416) (13.0062, 27.6539) (13.0077, 27.6661) (13.0092, 27.6785) (13.0107, 27.6908) (13.0122, 27.7032) (13.0136, 27.7157) (13.0151, 27.7281) (13.0165, 27.7406) (13.018, 27.7532) (13.0194, 27.7658) (13.0208, 27.7784) (13.0222, 27.791) (13.0236, 27.8037) (13.0249, 27.8164) (13.0263, 27.8291) (13.0276, 27.8419) (13.029, 27.8547) (13.0303, 27.8676) (13.0316, 27.8805) (13.0329, 27.8934) (13.0342, 27.9063) (13.0354, 27.9193) (13.0367, 27.9323) (13.0379, 27.9454) (13.0391, 27.9585) (13.0404, 27.9716) (13.0415, 27.9848) (13.0427, 27.9979) (13.0439, 28.0112) (13.0451, 28.0244) (13.0462, 28.0377) (13.0473, 28.051) (13.0484, 28.0644) (13.0495, 28.0777) (13.0506, 28.0911) (13.0515, 28.1019) (13.0521, 28.11) (13.0525, 28.1154) (13.0527, 28.1181) knots 0 0 0 0 0 0 0.00416667 0.00833333 0.0125 0.01666667 0.02083333 0.025 0.02916667 0.03333333 0.0375 0.04166667 0.04583333 0.05 0.05416667 0.05833333 0.0625 0.06666667 0.07083333 0.075 0.07916667 0.08333333 0.0875 0.09166667 0.09583333 0.1 0.10416667 0.10833333 0.1125 0.11666667 0.12083333 0.125 0.12916667 0.13333333 0.1375 0.14166667 0.14583333 0.15 0.15416667 0.15833333 0.1625 0.16666667 0.17083333 0.175 0.17916667 0.18333333 0.1875 0.19166667 0.19583333 0.2 0.20416667 0.20833333 0.2125 0.21666667 0.22083333 0.225 0.22916667 0.23333333 0.2375 0.24166667 0.24583333 0.25 0.25416667 0.25833333 0.2625 0.26666667 0.27083333 0.275 0.27916667 0.28333333 0.2875 0.29166667 0.29583333 0.3 0.30416667 0.30833333 0.3125 0.31666667 0.32083333 0.325 0.32916667 0.33333333 0.3375 0.34166667 0.34583333 0.35 0.35416667 0.35833333 0.3625 0.36666667 0.37083333 0.375 0.37916667 0.38333333 0.3875 0.39166667 0.39583333 0.4 0.40416667 0.40833333 0.4125 0.41666667 0.42083333 0.425 0.42916667 0.43333333 0.4375 0.44166667 0.44583333 0.45 0.45416667 0.45833333 0.4625 0.46666667 0.47083333 0.475 0.47916667 0.48333333 0.4875 0.49166667 0.49583333 0.5 0.50416667 0.50833333 0.5125 0.51666667 0.52083333 0.525 0.52916667 0.53333333 0.5375 0.54166667 0.54583333 0.55 0.55416667 0.55833333 0.5625 0.56666667 0.57083333 0.575 0.57916667 0.58333333 0.5875 0.59166667 0.59583333 0.6 0.60416667 0.60833333 0.6125 0.61666667 0.62083333 0.625 0.62916667 0.63333333 0.6375 0.64166667 0.64583333 0.65 0.65416667 0.65833333 0.6625 0.66666667 0.67083333 0.675 0.67916667 0.68333333 0.6875 0.69166667 0.69583333 0.7 0.70416667 0.70833333 0.7125 0.71666667 0.72083333 0.725 0.72916667 0.73333333 0.7375 0.74166667 0.74583333 0.75 0.75416667 0.75833333 0.7625 0.76666667 0.77083333 0.775 0.77916667 0.78333333 0.7875 0.79166667 0.79583333 0.8 0.80416667 0.80833333 0.8125 0.81666667 0.82083333 0.825 0.82916667 0.83333333 0.8375 0.84166667 0.84583333 0.85 0.85416667 0.85833333 0.8625 0.86666667 0.87083333 0.875 0.87916667 0.88333333 0.8875 0.89166667 0.89583333 0.9 0.90416667 0.90833333 0.9125 0.91666667 0.92083333 0.925 0.92916667 0.93333333 0.9375 0.94166667 0.94583333 0.95 0.95416667 0.95833333 0.9625 0.96666667 0.97083333 0.975 0.97916667 0.98333333 0.9875 0.99166667 0.99583333 1 1 1 1 1 1
  arc A89 (-28.6734, 2.0967) -> (-28.7355, 0.9119) centre (0, 0) ccw
  spline S88 degree 5 poles (9.8472, 27.3251) (9.8472, 27.3252) (9.8473, 27.3254) (9.8474, 27.3257) (9.8475, 27.3262) (9.8478, 27.3269) (9.8481, 27.3277) (9.8484, 27.3286) (9.8487, 27.3296) (9.8491, 27.3308) (9.8495, 27.332) (9.85, 27.3334) (9.8505, 27.3348) (9.851, 27.3364) (9.8515, 27.338) (9.8521, 27.3398) (9.8527, 27.3416) (9.8533, 27.3435) (9.8539, 27.3456) (9.8546, 27.3477) (9.8553, 27.3499) (9.856, 27.3523) (9.8568, 27.3547) (9.8575, 27.3572) (9.8583, 27.3598) (9.8591, 27.3625) (9.86, 27.3652) (9.8608, 27.3681) (9.8617, 27.371) (9.8626, 27.3741) (9.8635, 27.3772) (9.8645, 27.3804) (9.8654, 27.3837) (9.8664, 27.387) (9.8674, 27.3905) (9.8684, 27.394) (9.8694, 27.3976) (9.8704, 27.4013) (9.8715, 27.4051) (9.8725, 27.409) (9.8736, 27.4129) (9.8747, 27.4169) (9.8758, 27.421) (9.8769, 27.4252) (9.878, 27.4294) (9.8792, 27.4337) (9.8803, 27.4381) (9.8815, 27.4426) (9.8827, 27.4471) (9.8838, 27.4517) (9.885, 27.4564) (9.8862, 27.4612) (9.8874, 27.466) (9.8887, 27.4709) (9.8899, 27.4759) (9.8911, 27.481) (9.8924, 27.4861) (9.8936, 27.4912) (9.8949, 27.4965) (9.8962, 27.5018) (9.8974, 27.5072) (9.8987, 27.5127) (9.9, 27.5182) (9.9013, 27.5238) (9.9026, 27.5294) (9.9039, 27.5352) (9.9052, 27.5409) (9.9065, 27.5468) (9.9079, 27.5527) (9.9092, 27.5587) (9.9105, 27.5647) (9.9118, 27.5709) (9.9132, 27.577) (9.9145, 27.5833) (9.9158, 27.5896) (9.9172, 27.5959) (9.9185, 27.6023) (9.9199, 27.6088) (9.9212, 27.6154) (9.9225, 27.622) (9.9239, 27.6286) (9.9252, 27.6353) (9.9266, 27.6421) (9.9279, 27.649) (9.9293, 27.6559) (9.9306, 27.6628) (9.932, 27.6698) (9.9333, 27.6769) (9.9347, 27.6841) (9.936, 27.6912) (9.9374, 27.6985) (9.9387, 27.7058) (9.9401, 27.7132) (9.9414, 27.7206) (9.9428, 27.728) (9.9441, 27.7356) (9.9454, 27.7431) (9.9468, 27.7508) (9.9481, 27.7585) (9.9494, 27.7662) (9.9508, 27.774) (9.9521, 27.7819) (9.9534, 27.7898) (9.9547, 27.7977) (9.956, 27.8057) (9.9573, 27.8138) (9.9586, 27.8219) (9.9599, 27.8301) (9.9612, 27.8383) (9.9625, 27.8466) (9.9638, 27.8549) (9.9651, 27.8633) (9.9664, 27.8717) (9.9676, 27.8802) (9.9689, 27.8887) (9.9701, 27.8973) (9.9714, 27.9059) (9.9726, 27.9146) (9.9739, 27.9233) (9.9751, 27.9321) (9.9763, 27.9409) (9.9776, 27.9498) (9.9788, 27.9587) (9.98, 27.9677) (9.9812, 27.9767) (9.9824, 27.9858) (9.9836, 27.9949) (9.9847, 28.004) (9.9859, 28.0133) (9.9871, 28.0225) (9.9882, 28.0318) (9.9894, 28.0412) (9.9905, 28.0506) (9.9916, 28.06) (9.9928, 28.0695) (9.9939, 28.079) (9.995, 28.0886) (9.9961, 28.0982) (9.9972, 28.1079) (9.9983, 28.1176) (9.9993, 28.1274) (10.0004, 28.1372) (10.0014, 28.147) (10.0025, 28.1569) (10.0035, 28.1668) (10.0045, 28.1768) (10.0055, 28.1868) (10.0065, 28.1969) (10.0075, 28.207) (10.0085, 28.2172) (10.0095, 28.2274) (10.0104, 28.2376) (10.0114, 28.2479) (10.0123, 28.2582) (10.0133, 28.2686) (10.0142, 28.279) (10.0151, 28.2894) (10.016, 28.2999) (10.0169, 28.3105) (10.0177, 28.321) (10.0186, 28.3317) (10.0195, 28.3423) (10.0203, 28.353) (10.0211, 28.3638) (10.0219, 28.3745) (10.0227, 28.3854) (10.0235, 28.3962) (10.0243, 28.4071) (10.0251, 28.4181) (10.0258, 28.429) (10.0266, 28.44) (10.0273, 28.4511) (10.028, 28.4622) (10.0287, 28.4733) (10.0294, 28.4845) (10.0301, 28.4957) (10.0308, 28.507) (10.0314, 28.5183) (10.0321, 28.5296) (10.0327, 28.541) (10.0333, 28.5524) (10.0339, 28.5638) (10.0345, 28.5753) (10.0351, 28.5868) (10.0356, 28.5984) (10.0362, 28.61) (10.0367, 28.6216) (10.0372, 28.6333) (10.0377, 28.645) (10.0382, 28.6567) (10.0387, 28.6685) (10.0392, 28.6803) (10.0396, 28.6922) (10.04, 28.7041) (10.0405, 28.716) (10.0409, 28.728) (10.0412, 28.74) (10.0416, 28.752) (10.042, 28.7641) (10.0423, 28.7762) (10.0427, 28.7883) (10.043, 28.8005) (10.0433, 28.8127) (10.0436, 28.8249) (10.0438, 28.8372) (10.0441, 28.8495) (10.0443, 28.8619) (10.0445, 28.8743) (10.0448, 28.8867) (10.0449, 28.8991) (10.0451, 28.9116) (10.0453, 28.9241) (10.0454, 28.9367) (10.0456, 28.9493) (10.0457, 28.9619) (10.0458, 28.9745) (10.0458, 28.9872) (10.0459, 29) (10.046, 29.0127) (10.046, 29.0255) (10.046, 29.0383) (10.046, 29.0512) (10.046, 29.0641) (10.046, 29.077) (10.0459, 29.0899) (10.0458, 29.1029) (10.0458, 29.1159) (10.0457, 29.129) (10.0455, 29.142) (10.0454, 29.1551) (10.0453, 29.1683) (10.0451, 29.1815) (10.0449, 29.1947) (10.0447, 29.2079) (10.0445, 29.2212) (10.0442, 29.2345) (10.044, 29.2478) (10.0437, 29.2612) (10.0434, 29.2745) (10.0431, 29.288) (10.0428, 29.3014) (10.0425, 29.3122) (10.0423, 29.3203) (10.0422, 29.3257) (10.0421, 29.3284) knots 0 0 0 0 0 0 0.00416667 0.00833333 0.0125 0.01666667 0.02083333 0.025 0.02916667 0.03333333 0.0375 0.04166667 0.04583333 0.05 0.05416667 0.05833333 0.0625 0.06666667 0.07083333 0.075 0.07916667 0.08333333 0.0875 0.09166667 0.09583333 0.1 0.10416667 0.10833333 0.1125 0.11666667 0.12083333 0.125 0.12916667 0.13333333 0.1375 0.14166667 0.14583333 0.15 0.15416667 0.15833333 0.1625 0.16666667 0.17083333 0.175 0.17916667 0.18333333 0.1875 0.19166667 0.19583333 0.2 0.20416667 0.20833333 0.2125 0.21666667 0.22083333 0.225 0.22916667 0.23333333 0.2375 0.24166667 0.24583333 0.25 0.25416667 0.25833333 0.2625 0.26666667 0.27083333 0.275 0.27916667 0.28333333 0.2875 0.29166667 0.29583333 0.3 0.30416667 0.30833333 0.3125 0.31666667 0.32083333 0.325 0.32916667 0.33333333 0.3375 0.34166667 0.34583333 0.35 0.35416667 0.35833333 0.3625 0.36666667 0.37083333 0.375 0.37916667 0.38333333 0.3875 0.39166667 0.39583333 0.4 0.40416667 0.40833333 0.4125 0.41666667 0.42083333 0.425 0.42916667 0.43333333 0.4375 0.44166667 0.44583333 0.45 0.45416667 0.45833333 0.4625 0.46666667 0.47083333 0.475 0.47916667 0.48333333 0.4875 0.49166667 0.49583333 0.5 0.50416667 0.50833333 0.5125 0.51666667 0.52083333 0.525 0.52916667 0.53333333 0.5375 0.54166667 0.54583333 0.55 0.55416667 0.55833333 0.5625 0.56666667 0.57083333 0.575 0.57916667 0.58333333 0.5875 0.59166667 0.59583333 0.6 0.60416667 0.60833333 0.6125 0.61666667 0.62083333 0.625 0.62916667 0.63333333 0.6375 0.64166667 0.64583333 0.65 0.65416667 0.65833333 0.6625 0.66666667 0.67083333 0.675 0.67916667 0.68333333 0.6875 0.69166667 0.69583333 0.7 0.70416667 0.70833333 0.7125 0.71666667 0.72083333 0.725 0.72916667 0.73333333 0.7375 0.74166667 0.74583333 0.75 0.75416667 0.75833333 0.7625 0.76666667 0.77083333 0.775 0.77916667 0.78333333 0.7875 0.79166667 0.79583333 0.8 0.80416667 0.80833333 0.8125 0.81666667 0.82083333 0.825 0.82916667 0.83333333 0.8375 0.84166667 0.84583333 0.85 0.85416667 0.85833333 0.8625 0.86666667 0.87083333 0.875 0.87916667 0.88333333 0.8875 0.89166667 0.89583333 0.9 0.90416667 0.90833333 0.9125 0.91666667 0.92083333 0.925 0.92916667 0.93333333 0.9375 0.94166667 0.94583333 0.95 0.95416667 0.95833333 0.9625 0.96666667 0.97083333 0.975 0.97916667 0.98333333 0.9875 0.99166667 0.99583333 1 1 1 1 1 1
  line L184 (-28.9679, 2.1183) -> (-28.9671, 2.1182)
  spline S89 degree 5 poles (-30.8773, 2.755) (-30.8749, 2.7539) (-30.87, 2.7515) (-30.8627, 2.748) (-30.853, 2.7434) (-30.8408, 2.7376) (-30.8287, 2.7319) (-30.8165, 2.7262) (-30.8044, 2.7205) (-30.7924, 2.7149) (-30.7803, 2.7092) (-30.7683, 2.7036) (-30.7563, 2.6981) (-30.7443, 2.6925) (-30.7323, 2.687) (-30.7204, 2.6815) (-30.7085, 2.6761) (-30.6966, 2.6707) (-30.6847, 2.6653) (-30.6728, 2.6599) (-30.661, 2.6545) (-30.6492, 2.6492) (-30.6374, 2.6439) (-30.6256, 2.6387) (-30.6139, 2.6335) (-30.6022, 2.6283) (-30.5905, 2.6231) (-30.5788, 2.6179) (-30.5672, 2.6128) (-30.5555, 2.6077) (-30.5439, 2.6027) (-30.5324, 2.5977) (-30.5208, 2.5927) (-30.5093, 2.5877) (-30.4978, 2.5827) (-30.4863, 2.5778) (-30.4749, 2.5729) (-30.4634, 2.5681) (-30.452, 2.5632) (-30.4407, 2.5584) (-30.4293, 2.5537) (-30.418, 2.5489) (-30.4067, 2.5442) (-30.3954, 2.5395) (-30.3841, 2.5348) (-30.3729, 2.5302) (-30.3617, 2.5256) (-30.3506, 2.521) (-30.3394, 2.5165) (-30.3283, 2.5119) (-30.3172, 2.5074) (-30.3061, 2.503) (-30.2951, 2.4985) (-30.2841, 2.4941) (-30.2731, 2.4897) (-30.2621, 2.4854) (-30.2512, 2.481) (-30.2403, 2.4767) (-30.2294, 2.4725) (-30.2186, 2.4682) (-30.2078, 2.464) (-30.197, 2.4598) (-30.1862, 2.4557) (-30.1755, 2.4515) (-30.1648, 2.4474) (-30.1541, 2.4433) (-30.1435, 2.4393) (-30.1329, 2.4353) (-30.1223, 2.4313) (-30.1118, 2.4273) (-30.1012, 2.4234) (-30.0907, 2.4194) (-30.0803, 2.4156) (-30.0699, 2.4117) (-30.0595, 2.4079) (-30.0491, 2.4041) (-30.0388, 2.4003) (-30.0284, 2.3965) (-30.0182, 2.3928) (-30.0079, 2.3891) (-29.9977, 2.3855) (-29.9875, 2.3818) (-29.9774, 2.3782) (-29.9673, 2.3746) (-29.9572, 2.3711) (-29.9471, 2.3675) (-29.9371, 2.364) (-29.9271, 2.3606) (-29.9172, 2.3571) (-29.9073, 2.3537) (-29.8974, 2.3503) (-29.8875, 2.3469) (-29.8777, 2.3436) (-29.868, 2.3403) (-29.8582, 2.337) (-29.8485, 2.3337) (-29.8388, 2.3305) (-29.8292, 2.3273) (-29.8196, 2.3241) (-29.81, 2.321) (-29.8005, 2.3178) (-29.791, 2.3147) (-29.7815, 2.3117) (-29.7721, 2.3086) (-29.7627, 2.3056) (-29.7534, 2.3026) (-29.7441, 2.2996) (-29.7348, 2.2967) (-29.7255, 2.2938) (-29.7163, 2.2909) (-29.7072, 2.288) (-29.6981, 2.2852) (-29.689, 2.2824) (-29.6799, 2.2796) (-29.6709, 2.2769) (-29.6619, 2.2741) (-29.653, 2.2714) (-29.6441, 2.2688) (-29.6353, 2.2661) (-29.6265, 2.2635) (-29.6177, 2.2609) (-29.609, 2.2583) (-29.6003, 2.2558) (-29.5917, 2.2533) (-29.583, 2.2508) (-29.5745, 2.2483) (-29.566, 2.2458) (-29.5575, 2.2434) (-29.5491, 2.241) (-29.5407, 2.2387) (-29.5323, 2.2363) (-29.524, 2.234) (-29.5158, 2.2317) (-29.5075, 2.2295) (-29.4994, 2.2272) (-29.4912, 2.225) (-29.4832, 2.2228) (-29.4751, 2.2207) (-29.4671, 2.2185) (-29.4592, 2.2164) (-29.4513, 2.2143) (-29.4434, 2.2123) (-29.4356, 2.2102) (-29.4279, 2.2082) (-29.4202, 2.2062) (-29.4125, 2.2043) (-29.4049, 2.2023) (-29.3973, 2.2004) (-29.3898, 2.1985) (-29.3823, 2.1967) (-29.3749, 2.1948) (-29.3675, 2.193) (-29.3602, 2.1912) (-29.3529, 2.1895) (-29.3457, 2.1877) (-29.3386, 2.186) (-29.3314, 2.1843) (-29.3244, 2.1827) (-29.3174, 2.181) (-29.3104, 2.1794) (-29.3035, 2.1778) (-29.2967, 2.1762) (-29.2899, 2.1747) (-29.2831, 2.1731) (-29.2764, 2.1716) (-29.2698, 2.1702) (-29.2632, 2.1687) (-29.2567, 2.1673) (-29.2502, 2.1659) (-29.2438, 2.1645) (-29.2374, 2.1631) (-29.2311, 2.1618) (-29.2249, 2.1605) (-29.2187, 2.1592) (-29.2126, 2.1579) (-29.2065, 2.1567) (-29.2005, 2.1554) (-29.1946, 2.1542) (-29.1887, 2.153) (-29.1829, 2.1519) (-29.1771, 2.1507) (-29.1714, 2.1496) (-29.1658, 2.1485) (-29.1602, 2.1475) (-29.1547, 2.1464) (-29.1493, 2.1454) (-29.1439, 2.1444) (-29.1386, 2.1434) (-29.1334, 2.1424) (-29.1282, 2.1415) (-29.1231, 2.1406) (-29.118, 2.1397) (-29.1131, 2.1388) (-29.1081, 2.138) (-29.1033, 2.1371) (-29.0985, 2.1363) (-29.0938, 2.1355) (-29.0892, 2.1347) (-29.0847, 2.134) (-29.0802, 2.1332) (-29.0758, 2.1325) (-29.0714, 2.1318) (-29.0672, 2.1312) (-29.063, 2.1305) (-29.0589, 2.1299) (-29.0549, 2.1292) (-29.0509, 2.1286) (-29.047, 2.1281) (-29.0432, 2.1275) (-29.0395, 2.127) (-29.0359, 2.1264) (-29.0323, 2.1259) (-29.0289, 2.1254) (-29.0255, 2.125) (-29.0222, 2.1245) (-29.0189, 2.1241) (-29.0158, 2.1237) (-29.0128, 2.1233) (-29.0098, 2.1229) (-29.0069, 2.1225) (-29.0041, 2.1222) (-29.0015, 2.1219) (-28.9989, 2.1215) (-28.9963, 2.1212) (-28.9939, 2.121) (-28.9916, 2.1207) (-28.9894, 2.1204) (-28.9873, 2.1202) (-28.9852, 2.12) (-28.9833, 2.1198) (-28.9815, 2.1196) (-28.9798, 2.1194) (-28.9781, 2.1192) (-28.9766, 2.1191) (-28.9752, 2.1189) (-28.9739, 2.1188) (-28.9727, 2.1187) (-28.9716, 2.1186) (-28.9706, 2.1185) (-28.9698, 2.1184) (-28.969, 2.1184) (-28.9685, 2.1183) (-28.9682, 2.1183) (-28.968, 2.1183) (-28.9679, 2.1183) knots -1 -1 -1 -1 -1 -1 -0.99583333 -0.99166667 -0.9875 -0.98333333 -0.97916667 -0.975 -0.97083333 -0.96666667 -0.9625 -0.95833333 -0.95416667 -0.95 -0.94583333 -0.94166667 -0.9375 -0.93333333 -0.92916667 -0.925 -0.92083333 -0.91666667 -0.9125 -0.90833333 -0.90416667 -0.9 -0.89583333 -0.89166667 -0.8875 -0.88333333 -0.87916667 -0.875 -0.87083333 -0.86666667 -0.8625 -0.85833333 -0.85416667 -0.85 -0.84583333 -0.84166667 -0.8375 -0.83333333 -0.82916667 -0.825 -0.82083333 -0.81666667 -0.8125 -0.80833333 -0.80416667 -0.8 -0.79583333 -0.79166667 -0.7875 -0.78333333 -0.77916667 -0.775 -0.77083333 -0.76666667 -0.7625 -0.75833333 -0.75416667 -0.75 -0.74583333 -0.74166667 -0.7375 -0.73333333 -0.72916667 -0.725 -0.72083333 -0.71666667 -0.7125 -0.70833333 -0.70416667 -0.7 -0.69583333 -0.69166667 -0.6875 -0.68333333 -0.67916667 -0.675 -0.67083333 -0.66666667 -0.6625 -0.65833333 -0.65416667 -0.65 -0.64583333 -0.64166667 -0.6375 -0.63333333 -0.62916667 -0.625 -0.62083333 -0.61666667 -0.6125 -0.60833333 -0.60416667 -0.6 -0.59583333 -0.59166667 -0.5875 -0.58333333 -0.57916667 -0.575 -0.57083333 -0.56666667 -0.5625 -0.55833333 -0.55416667 -0.55 -0.54583333 -0.54166667 -0.5375 -0.53333333 -0.52916667 -0.525 -0.52083333 -0.51666667 -0.5125 -0.50833333 -0.50416667 -0.5 -0.49583333 -0.49166667 -0.4875 -0.48333333 -0.47916667 -0.475 -0.47083333 -0.46666667 -0.4625 -0.45833333 -0.45416667 -0.45 -0.44583333 -0.44166667 -0.4375 -0.43333333 -0.42916667 -0.425 -0.42083333 -0.41666667 -0.4125 -0.40833333 -0.40416667 -0.4 -0.39583333 -0.39166667 -0.3875 -0.38333333 -0.37916667 -0.375 -0.37083333 -0.36666667 -0.3625 -0.35833333 -0.35416667 -0.35 -0.34583333 -0.34166667 -0.3375 -0.33333333 -0.32916667 -0.325 -0.32083333 -0.31666667 -0.3125 -0.30833333 -0.30416667 -0.3 -0.29583333 -0.29166667 -0.2875 -0.28333333 -0.27916667 -0.275 -0.27083333 -0.26666667 -0.2625 -0.25833333 -0.25416667 -0.25 -0.24583333 -0.24166667 -0.2375 -0.23333333 -0.22916667 -0.225 -0.22083333 -0.21666667 -0.2125 -0.20833333 -0.20416667 -0.2 -0.19583333 -0.19166667 -0.1875 -0.18333333 -0.17916667 -0.175 -0.17083333 -0.16666667 -0.1625 -0.15833333 -0.15416667 -0.15 -0.14583333 -0.14166667 -0.1375 -0.13333333 -0.12916667 -0.125 -0.12083333 -0.11666667 -0.1125 -0.10833333 -0.10416667 -0.1 -0.09583333 -0.09166667 -0.0875 -0.08333333 -0.07916667 -0.075 -0.07083333 -0.06666667 -0.0625 -0.05833333 -0.05416667 -0.05 -0.04583333 -0.04166667 -0.0375 -0.03333333 -0.02916667 -0.025 -0.02083333 -0.01666667 -0.0125 -0.00833333 -0.00416667 0 0 0 0 0 0
  spline S90 degree 5 poles (6.937, 28.2047) (6.937, 28.2048) (6.937, 28.205) (6.9371, 28.2053) (6.9372, 28.2058) (6.9374, 28.2065) (6.9376, 28.2074) (6.9378, 28.2083) (6.9381, 28.2094) (6.9383, 28.2106) (6.9386, 28.2118) (6.9389, 28.2132) (6.9392, 28.2147) (6.9396, 28.2163) (6.9399, 28.218) (6.9403, 28.2198) (6.9407, 28.2217) (6.9411, 28.2237) (6.9416, 28.2258) (6.942, 28.228) (6.9425, 28.2303) (6.9429, 28.2327) (6.9434, 28.2351) (6.9439, 28.2377) (6.9445, 28.2404) (6.945, 28.2431) (6.9455, 28.246) (6.9461, 28.2489) (6.9466, 28.2519) (6.9472, 28.255) (6.9478, 28.2582) (6.9484, 28.2615) (6.949, 28.2649) (6.9496, 28.2683) (6.9502, 28.2719) (6.9508, 28.2755) (6.9515, 28.2792) (6.9521, 28.283) (6.9528, 28.2868) (6.9534, 28.2908) (6.9541, 28.2948) (6.9547, 28.2989) (6.9554, 28.3031) (6.9561, 28.3074) (6.9568, 28.3117) (6.9574, 28.3161) (6.9581, 28.3206) (6.9588, 28.3252) (6.9595, 28.3298) (6.9602, 28.3345) (6.9609, 28.3393) (6.9616, 28.3442) (6.9623, 28.3491) (6.963, 28.3541) (6.9637, 28.3592) (6.9644, 28.3643) (6.9651, 28.3695) (6.9658, 28.3748) (6.9665, 28.3802) (6.9672, 28.3856) (6.9679, 28.3911) (6.9686, 28.3966) (6.9693, 28.4023) (6.97, 28.408) (6.9707, 28.4137) (6.9714, 28.4196) (6.9721, 28.4255) (6.9728, 28.4314) (6.9735, 28.4374) (6.9742, 28.4435) (6.9749, 28.4497) (6.9756, 28.4559) (6.9763, 28.4622) (6.9769, 28.4685) (6.9776, 28.4749) (6.9783, 28.4814) (6.9789, 28.4879) (6.9796, 28.4945) (6.9803, 28.5011) (6.9809, 28.5078) (6.9816, 28.5146) (6.9822, 28.5214) (6.9828, 28.5283) (6.9835, 28.5353) (6.9841, 28.5423) (6.9847, 28.5493) (6.9853, 28.5564) (6.9859, 28.5636) (6.9865, 28.5709) (6.9871, 28.5781) (6.9877, 28.5855) (6.9882, 28.5929) (6.9888, 28.6004) (6.9894, 28.6079) (6.9899, 28.6154) (6.9905, 28.6231) (6.991, 28.6307) (6.9915, 28.6385) (6.9921, 28.6463) (6.9926, 28.6541) (6.9931, 28.662) (6.9936, 28.67) (6.994, 28.678) (6.9945, 28.686) (6.995, 28.6941) (6.9954, 28.7023) (6.9959, 28.7105) (6.9963, 28.7187) (6.9968, 28.727) (6.9972, 28.7354) (6.9976, 28.7438) (6.998, 28.7523) (6.9984, 28.7608) (6.9987, 28.7694) (6.9991, 28.778) (6.9995, 28.7866) (6.9998, 28.7953) (7.0001, 28.8041) (7.0005, 28.8129) (7.0008, 28.8218) (7.0011, 28.8307) (7.0014, 28.8396) (7.0016, 28.8486) (7.0019, 28.8577) (7.0021, 28.8668) (7.0024, 28.8759) (7.0026, 28.8851) (7.0028, 28.8943) (7.003, 28.9036) (7.0032, 28.9129) (7.0034, 28.9223) (7.0036, 28.9317) (7.0037, 28.9412) (7.0038, 28.9507) (7.004, 28.9602) (7.0041, 28.9698) (7.0042, 28.9795) (7.0043, 28.9892) (7.0043, 28.9989) (7.0044, 29.0087) (7.0044, 29.0185) (7.0045, 29.0284) (7.0045, 29.0383) (7.0045, 29.0482) (7.0045, 29.0582) (7.0044, 29.0682) (7.0044, 29.0783) (7.0043, 29.0884) (7.0043, 29.0986) (7.0042, 29.1088) (7.0041, 29.119) (7.004, 29.1293) (7.0038, 29.1396) (7.0037, 29.15) (7.0035, 29.1604) (7.0034, 29.1708) (7.0032, 29.1813) (7.003, 29.1919) (7.0028, 29.2024) (7.0025, 29.213) (7.0023, 29.2237) (7.002, 29.2344) (7.0017, 29.2451) (7.0014, 29.2559) (7.0011, 29.2667) (7.0008, 29.2775) (7.0004, 29.2884) (7.0001, 29.2993) (6.9997, 29.3103) (6.9993, 29.3213) (6.9989, 29.3323) (6.9984, 29.3434) (6.998, 29.3545) (6.9975, 29.3657) (6.997, 29.3768) (6.9965, 29.3881) (6.996, 29.3993) (6.9955, 29.4106) (6.995, 29.422) (6.9944, 29.4333) (6.9938, 29.4447) (6.9932, 29.4562) (6.9926, 29.4677) (6.992, 29.4792) (6.9913, 29.4907) (6.9906, 29.5023) (6.99, 29.514) (6.9892, 29.5256) (6.9885, 29.5373) (6.9878, 29.549) (6.987, 29.5608) (6.9863, 29.5726) (6.9855, 29.5844) (6.9846, 29.5963) (6.9838, 29.6082) (6.983, 29.6201) (6.9821, 29.6321) (6.9812, 29.6441) (6.9803, 29.6562) (6.9794, 29.6682) (6.9784, 29.6803) (6.9775, 29.6925) (6.9765, 29.7047) (6.9755, 29.7169) (6.9745, 29.7291) (6.9735, 29.7414) (6.9724, 29.7537) (6.9713, 29.766) (6.9702, 29.7784) (6.9691, 29.7908) (6.968, 29.8032) (6.9669, 29.8157) (6.9657, 29.8282) (6.9645, 29.8407) (6.9633, 29.8533) (6.9621, 29.8659) (6.9608, 29.8785) (6.9596, 29.8912) (6.9583, 29.9039) (6.957, 29.9166) (6.9556, 29.9293) (6.9543, 29.9421) (6.9529, 29.9549) (6.9516, 29.9678) (6.9501, 29.9806) (6.9487, 29.9935) (6.9473, 30.0065) (6.9458, 30.0194) (6.9443, 30.0324) (6.9428, 30.0455) (6.9413, 30.0585) (6.9398, 30.0716) (6.9382, 30.0847) (6.9366, 30.0979) (6.935, 30.111) (6.9334, 30.1242) (6.9317, 30.1375) (6.9301, 30.1507) (6.9284, 30.164) (6.9267, 30.1773) (6.925, 30.1907) (6.9236, 30.2014) (6.9225, 30.2094) (6.9218, 30.2148) (6.9214, 30.2174) knots 0 0 0 0 0 0 0.00416667 0.00833333 0.0125 0.01666667 0.02083333 0.025 0.02916667 0.03333333 0.0375 0.04166667 0.04583333 0.05 0.05416667 0.05833333 0.0625 0.06666667 0.07083333 0.075 0.07916667 0.08333333 0.0875 0.09166667 0.09583333 0.1 0.10416667 0.10833333 0.1125 0.11666667 0.12083333 0.125 0.12916667 0.13333333 0.1375 0.14166667 0.14583333 0.15 0.15416667 0.15833333 0.1625 0.16666667 0.17083333 0.175 0.17916667 0.18333333 0.1875 0.19166667 0.19583333 0.2 0.20416667 0.20833333 0.2125 0.21666667 0.22083333 0.225 0.22916667 0.23333333 0.2375 0.24166667 0.24583333 0.25 0.25416667 0.25833333 0.2625 0.26666667 0.27083333 0.275 0.27916667 0.28333333 0.2875 0.29166667 0.29583333 0.3 0.30416667 0.30833333 0.3125 0.31666667 0.32083333 0.325 0.32916667 0.33333333 0.3375 0.34166667 0.34583333 0.35 0.35416667 0.35833333 0.3625 0.36666667 0.37083333 0.375 0.37916667 0.38333333 0.3875 0.39166667 0.39583333 0.4 0.40416667 0.40833333 0.4125 0.41666667 0.42083333 0.425 0.42916667 0.43333333 0.4375 0.44166667 0.44583333 0.45 0.45416667 0.45833333 0.4625 0.46666667 0.47083333 0.475 0.47916667 0.48333333 0.4875 0.49166667 0.49583333 0.5 0.50416667 0.50833333 0.5125 0.51666667 0.52083333 0.525 0.52916667 0.53333333 0.5375 0.54166667 0.54583333 0.55 0.55416667 0.55833333 0.5625 0.56666667 0.57083333 0.575 0.57916667 0.58333333 0.5875 0.59166667 0.59583333 0.6 0.60416667 0.60833333 0.6125 0.61666667 0.62083333 0.625 0.62916667 0.63333333 0.6375 0.64166667 0.64583333 0.65 0.65416667 0.65833333 0.6625 0.66666667 0.67083333 0.675 0.67916667 0.68333333 0.6875 0.69166667 0.69583333 0.7 0.70416667 0.70833333 0.7125 0.71666667 0.72083333 0.725 0.72916667 0.73333333 0.7375 0.74166667 0.74583333 0.75 0.75416667 0.75833333 0.7625 0.76666667 0.77083333 0.775 0.77916667 0.78333333 0.7875 0.79166667 0.79583333 0.8 0.80416667 0.80833333 0.8125 0.81666667 0.82083333 0.825 0.82916667 0.83333333 0.8375 0.84166667 0.84583333 0.85 0.85416667 0.85833333 0.8625 0.86666667 0.87083333 0.875 0.87916667 0.88333333 0.8875 0.89166667 0.89583333 0.9 0.90416667 0.90833333 0.9125 0.91666667 0.92083333 0.925 0.92916667 0.93333333 0.9375 0.94166667 0.94583333 0.95 0.95416667 0.95833333 0.9625 0.96666667 0.97083333 0.975 0.97916667 0.98333333 0.9875 0.99166667 0.99583333 1 1 1 1 1 1
  line L185 (5.1346, 28.5878) -> (5.1345, 28.587)
  line L186 (-26.8948, 10.9659) -> (-26.6221, 10.8547)